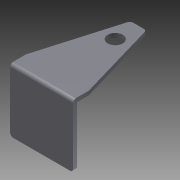
# Autodesk Inventor part: Control_Horn
Saved by Autodesk Inventor 2011 SP1 (Build 150282100, 282)
## iProperties
Created: 2011-06-11
Part Number: Control_Horn
Document SubType Name: Modeling
Designer: Andrew G. Meyer
Mass: 0.031742 g
Surface Area: 1.74038 cm^2
Volume: 0.031742 cm^3
Density: 1 g/cm^3
Author: Andrew G. Meyer
Autodesk Inventor part; units mm, degrees
ref_plane "YZ Plane" through (0, 0, 0) normal (1, 0, 0) x (0, 1, 0)
ref_plane "XZ Plane" through (0, 0, 0) normal (0, 1, 0) x (-1, 0, 0)
ref_plane "XY Plane" through (0, 0, 0) normal (0, 0, 1) x (1, 0, 0)
sketch "Sketch1" plane through (0, 0, 0) normal (0, 0, 1) x (1, 0, 0)
  line L0 (-3.175, 3.175) -> (3.175, 3.175)
  line L1 (3.175, 3.175) -> (3.175, -3.175)
  line L2 (3.175, -3.175) -> (-3.175, -3.175)
  line L3 (-3.175, -3.175) -> (-3.175, 3.175)
  point P0 (0, 0)
  dimension "d0" = 6.35
  dimension "d1" = 3.175
  dimension "d2" = 3.175
  constraints: 8 end point, 2 parallel, 2 perpendicular, 1 horizontal
  measures "d0" distance of L0.start L0.end
  measures "d1" distance from line of L0 point (0, 0)
  measures "d2" distance from line of L3 point (0, 0)
extrude "Extrusion1" add sketch "Sketch1" along normal blind 0.4064
sketch "Sketch2" plane through (-3.175, 3.175, 0) normal (0, 1, 0) x (1, 0, 0)
  line L0 (0, -0.4064) -> (6.35, -0.4064) projected
  line L1 (6.35, 0) -> (6.35, -0.4064) projected
  line L2 (0, 0) -> (6.35, 0) projected
  line L3 (0, 0) -> (0, -0.4064) projected
  line L4 (0, -0.4064) -> (6.35, -0.4064)
  line L5 (6.35, -0.4064) -> (6.35, 1.1811)
  line L6 (3.9688, 9.3726) -> (2.3812, 9.3726)
  line L7 (0, 1.1811) -> (0, -0.4064)
  line L8 (2.3812, 9.3726) -> (0, 1.1811)
  line L9 (3.9688, 9.3726) -> (6.35, 1.1811)
  point P0 (3.175, 0)
  dimension "d7" = 9.779
  dimension "d8" = 1.5875
  dimension "d9" = 1.5875
  constraints: 12 end point, 2 equal length, 2 parallel, 1 collinear, 1 horizontal, 1 perpendicular
  measures "d7" distance between parallel lines of L0 L6
  measures "d8" distance of L4.end L5.end
  measures "d9" distance of L6.start L6.end
extrude "Extrusion2" add sketch "Sketch2" against normal blind 0.4064 contours L7 L8 L6 L9 L5 L2
fillet "Fillet1" radius 0.3175 1 edges at (0, 3.175, 0.4064)
fillet "Fillet2" radius 0.3175 2 edges at (-0.7938, 2.9718, -9.3726) (0.7938, 2.9718, -9.3726)
fillet "Fillet3" radius 0.3175 4 edges at (3.175, -3.175, 0.2032) (-3.175, -3.175, 0.2032) (3.175, 2.9718, -1.1811) (-3.175, 2.9718, -1.1811)
hole "Hole1" at (0, 3.175, -7.0358) direction (0, -1, 0) diameter 1.524 depth 25.4 tip angle 118
equation "\"d1\" = 0.5 * d0"
equation "\"d2\" = d1"
body "Solid1"
